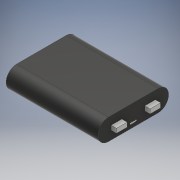
# Autodesk Inventor part: learnbot bateria
Saved by Autodesk Inventor 2017 (Build 210142000, 142)
## iProperties
Part Number: learnbot bateria
Material: Genérico
Document SubType Name: Modeling
Designer: rober
Density: 1 g/cm^3
Appearance: Valor por defecto
Author: rober
Autodesk Inventor part; units mm, degrees
ref_plane "YZ Plane" through (0, 0, 0) normal (1, 0, 0) x (0, 1, 0)
ref_plane "XZ Plane" through (0, 0, 0) normal (0, 1, 0) x (-1, 0, 0)
ref_plane "XY Plane" through (0, 0, 0) normal (0, 0, 1) x (1, 0, 0)
sketch "Boceto1" plane through (0, 0, 0) normal (0, 0, 1) x (1, 0, 0)
  line L0 (0, 0) -> (10.4, 0)
  line L1 (10.4, 0) -> (10.4, 8)
  line L2 (10.4, 8) -> (0, 8)
  line L3 (0, 8) -> (0, 0)
  line L4 (-0.6, 6.5) -> (0, 6.5)
  line L5 (-0.6, 6.5) -> (-0.6, 5.3)
  line L6 (-0.6, 5.3) -> (0, 5.3)
  line L7 (-0.6, 1.5) -> (0, 1.5)
  line L8 (-0.6, 1.5) -> (-0.6, 2.7)
  line L9 (-0.6, 2.7) -> (0, 2.7)
  line L10 (27.9808, 14.8149) -> (27.9808, 16.7149)
  line L11 (27.9808, 16.7149) -> (29.6808, 16.7149)
  line L12 (29.6808, 16.7149) -> (29.6808, 14.8149)
  line L13 (29.6808, 14.8149) -> (27.9808, 14.8149)
  line L14 (27.9808, 14.8149) -> (26.8808, 14.8149)
  line L15 (26.8808, 14.8149) -> (26.8808, 15.8149)
  line L16 (26.8808, 15.8149) -> (27.9808, 15.8149)
  line L17 (29.6808, 14.8149) -> (30.7808, 14.8149)
  line L18 (30.7808, 14.8149) -> (30.7808, 15.8149)
  line L19 (30.7808, 15.8149) -> (29.6808, 15.8149)
  circle A0 centre (27.4308, 15.3149) radius 0.15
  circle A1 centre (30.2308, 15.3149) radius 0.15
  constraints: 40 end point, 6 point on line, 2 centre point
extrude "Extrusión1" add sketch "Boceto1" along normal blind 2.4 contours L3 L2 L1 L0
sketch "Boceto2" plane through (10.4, 0, 0) normal (1, 0, 0) x (0, 0, -1)
  line L0 (0, 6.8) -> (0, 1.2)
  line L1 (-2.4, 6.8) -> (-2.4, 1.2)
  line L2 (-1.2, 1.5) -> (-1.45, 1.5)
  line L3 (-1.2, 1.5) -> (-0.95, 1.5)
  line L4 (-1.45, 6.5) -> (-0.95, 6.5)
  line L5 (-0.95, 6.5) -> (-0.95, 5.3)
  line L6 (-0.95, 5.3) -> (-1.45, 5.3)
  line L7 (-1.45, 5.3) -> (-1.45, 6.5)
  line L8 (-1.45, 2.7) -> (-0.95, 2.7)
  line L9 (-0.95, 2.7) -> (-0.95, 1.5)
  line L10 (-0.95, 1.5) -> (-1.45, 1.5)
  line L11 (-1.45, 1.5) -> (-1.45, 2.7)
  line L12 (-0.6, 3.6) -> (-0.5, 3.6)
  line L13 (-0.4, 3.7) -> (-0.5, 3.6)
  line L14 (-0.6, 3.6) -> (-0.6, 4.4)
  line L15 (-0.6, 4.4) -> (-0.5, 4.4)
  line L16 (-0.4, 4.3) -> (-0.5, 4.4)
  line L17 (-0.4, 4.3) -> (-0.4, 3.7)
  arc A0 (0, 6.8) -> (-2.4, 6.8) centre (-1.2, 6.8) ccw
  arc A1 (-2.4, 1.2) -> (0, 1.2) centre (-1.2, 1.2) ccw
  line L18 (0, 0) -> (0, 8) projected
  line L19 (0, 8) -> (-2.4, 8) projected
  line L20 (-2.4, 0) -> (-2.4, 8) projected
  line L21 (0, 0) -> (-2.4, 0) projected
  line L22 (-2.4, 0) -> (-2.4, 8) projected
  line L23 (-2.4, 1.2) -> (-2.4, 0)
  line L24 (0, 0) -> (-2.4, 0) projected
  line L25 (0, 0) -> (0, 1.2)
  line L26 (0, 0) -> (-2.4, 0)
  line L27 (-2.4, 6.8) -> (-2.4, 8)
  line L28 (-2.4, 8) -> (0, 8)
  line L29 (0, 8) -> (0, 6.8)
  line L30 (0, 0) -> (0, 8) projected
  constraints: 48 end point, 4 point on circle, 3 collinear, 3 perpendicular, 2 centre point, 2 tangent, 1 midpoint
extrude "Extrusión2" cut sketch "Boceto2" against normal blind 12.4 contours A0 L19 L18 | L18 L21 A1 | A0 L20 L19 | L21 L20 A1
sketch "Boceto3" plane through (10.4, 1.2, 0) normal (1, 0, 0) x (0, 0, -1)
  line L0 (0, 5.6) -> (0, 0)
  line L1 (-2.4, 5.6) -> (-2.4, 0)
  line L2 (-1.2, 0.3) -> (-1.45, 0.3)
  line L3 (-1.2, 0.3) -> (-0.95, 0.3)
  line L4 (-1.45, 5.3) -> (-0.95, 5.3)
  line L5 (-0.95, 5.3) -> (-0.95, 4.1)
  line L6 (-0.95, 4.1) -> (-1.45, 4.1)
  line L7 (-1.45, 4.1) -> (-1.45, 5.3)
  line L8 (-1.45, 1.5) -> (-0.95, 1.5)
  line L9 (-0.95, 1.5) -> (-0.95, 0.3)
  line L10 (-0.95, 0.3) -> (-1.45, 0.3)
  line L11 (-1.45, 0.3) -> (-1.45, 1.5)
  line L12 (-0.6, 2.4) -> (-0.5, 2.4)
  line L13 (-0.4, 2.5) -> (-0.5, 2.4)
  line L14 (-0.6, 2.4) -> (-0.6, 3.2)
  line L15 (-0.6, 3.2) -> (-0.5, 3.2)
  line L16 (-0.4, 3.1) -> (-0.5, 3.2)
  line L17 (-0.4, 3.1) -> (-0.4, 2.5)
  arc A0 (0, 5.6) -> (-2.4, 5.6) centre (-1.2, 5.6) ccw
  arc A1 (-2.4, 0) -> (0, 0) centre (-1.2, 0) ccw
  line L18 (0, -1.2) -> (0, 6.8)
  line L19 (0, 6.8) -> (-2.4, 6.8)
  line L20 (-2.4, -1.2) -> (-2.4, 6.8)
  line L21 (0, -1.2) -> (-2.4, -1.2)
  line L22 (-2.4, -1.2) -> (-2.4, 6.8)
  line L23 (-2.4, 0) -> (-2.4, -1.2)
  line L24 (0, -1.2) -> (-2.4, -1.2)
  line L25 (0, -1.2) -> (0, 0)
  line L26 (0, -1.2) -> (-2.4, -1.2)
  line L27 (-2.4, 5.6) -> (-2.4, 6.8)
  line L28 (-2.4, 6.8) -> (0, 6.8)
  line L29 (0, 6.8) -> (0, 5.6)
  line L30 (0, -1.2) -> (0, 6.8)
  constraints: 62 end point, 4 point on circle, 3 collinear, 3 perpendicular, 2 centre point, 2 tangent, 1 midpoint
extrude "Extrusión3" add sketch "Boceto3" along normal blind 0.6 contours L2 L11 L8 L9 L3 | L4 L5 L6 L7
sketch "Boceto4" plane through (10.4, 1.2, 0) normal (1, 0, 0) x (0, 0, -1)
  line L0 (-0.95, 5.3) -> (-0.95, 4.1)
  line L1 (-0.95, 4.1) -> (-1.45, 4.1)
  line L2 (-1.45, 4.1) -> (-1.45, 5.3)
  line L3 (-0.6, 3.2) -> (-0.5, 3.2)
  line L4 (-0.4, 3.1) -> (-0.5, 3.2)
  line L5 (0, -1.2) -> (0, 6.8)
  line L6 (0, -1.2) -> (0, 6.8)
  line L7 (-2.4, -1.2) -> (-2.4, 6.8)
  line L8 (-2.4, -1.2) -> (-2.4, 6.8)
  line L9 (-2.4, 5.6) -> (-2.4, 0)
  line L10 (0, 5.6) -> (0, 0)
  line L11 (-0.4, 3.1) -> (-0.4, 2.5)
  line L12 (-0.6, 2.4) -> (-0.6, 3.2)
  line L13 (-0.6, 2.4) -> (-0.5, 2.4)
  line L14 (-1.2, 0.3) -> (-1.45, 0.3)
  line L15 (-1.2, 0.3) -> (-0.95, 0.3)
  line L16 (-1.45, 1.5) -> (-0.95, 1.5)
  line L17 (-0.95, 1.5) -> (-0.95, 0.3)
  line L18 (-1.45, 0.3) -> (-1.45, 1.5)
  line L19 (-0.95, 0.3) -> (-1.45, 0.3)
  line L20 (0, -1.2) -> (0, 0)
  line L21 (-2.4, 0) -> (-2.4, -1.2)
  line L22 (0, -1.2) -> (-2.4, -1.2)
  line L23 (0, -1.2) -> (-2.4, -1.2)
  line L24 (0, -1.2) -> (-2.4, -1.2)
  arc A0 (-2.4, 0) -> (0, 0) centre (-1.2, 0) ccw
  line L25 (0, 6.8) -> (0, 5.6)
  line L26 (0, 6.8) -> (-2.4, 6.8)
  line L27 (-2.4, 6.8) -> (0, 6.8)
  arc A1 (0, 5.6) -> (-2.4, 5.6) centre (-1.2, 5.6) ccw
  line L28 (-2.4, 5.6) -> (-2.4, 6.8)
  line L29 (-1.45, 5.3) -> (-0.95, 5.3)
  line L30 (-0.4, 2.5) -> (-0.5, 2.4)
  constraints: 62 end point, 4 point on circle, 3 collinear, 3 perpendicular, 2 centre point, 2 tangent, 1 midpoint
extrude "Extrusión4" cut sketch "Boceto4" against normal blind 0.3 contours L3 L4 L11 L30 L13 L12
